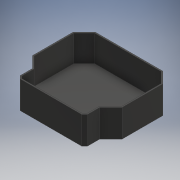
# Autodesk Inventor part: XT-SM-05
Saved by Autodesk Inventor 2017 (Build 210142000, 142)
## iProperties
Created: 2019-11-11
Part Number: XT-SM-05
Material: ABS Plastic
Document SubType Name: Modeling
Designer: Dell
Density: 1.06 g/cm^3
Appearance: Smooth - Black
Author: Dell
Autodesk Inventor part; units mm, degrees
ref_plane "YZ Plane" through (0, 0, 0) normal (1, 0, 0) x (0, 1, 0)
ref_plane "XZ Plane" through (0, 0, 0) normal (0, 1, 0) x (-1, 0, 0)
ref_plane "XY Plane" through (0, 0, 0) normal (0, 0, 1) x (1, 0, 0)
sketch "Sketch1" plane through (0, 0, 0) normal (0, 0, 1) x (1, 0, 0)
  line L0 (60.1273, -75.5) -> (55.1273, -80.5)
  line L1 (60.1273, -53.5) -> (60.1273, -75.5)
  line L2 (60.1273, -53.5) -> (80.1273, -33.5)
  line L3 (80.1273, 39) -> (80.1273, -33.5)
  line L4 (60.1273, 59) -> (80.1273, 39)
  line L5 (-60.1273, 59) -> (60.1273, 59)
  line L6 (-60.1273, 59) -> (-80.1273, 39)
  line L7 (-80.1273, 39) -> (-80.1273, -33.5)
  line L8 (-80.1273, -33.5) -> (-60.1273, -53.5)
  line L9 (-60.1273, -75.5) -> (-60.1273, -53.5)
  line L10 (-55.1273, -80.5) -> (-60.1273, -75.5)
  line L11 (55.1273, -80.5) -> (-55.1273, -80.5)
  point P0 (0, 0)
  point P1 (0, 0)
  point P2 (0, 59)
  dimension "d0" = 120.2547
  dimension "d1" = 72.5
  dimension "d2" = 22
  dimension "d3" = 110.2547
  dimension "d4" = 22
  dimension "d5" = 72.5
  dimension "d6" = 160.2547
  dimension "d7" = 139.5
  dimension "d8" = 27
  dimension "d9" = 27
  dimension "d10" = 20
  dimension "d11" = 20
  dimension "d12" = 20
  dimension "d14" = 20
  dimension "d15" = 20
  dimension "d16" = 5
  dimension "d17" = 20
  dimension "d18" = 59
  dimension "d19" = 80.1273
  constraints: 24 end point, 3 vertical, 1 coincident, 1 midpoint, 1 vertical alignment
  measures "d0" distance of L5.start L5.end
  measures "d1" distance of L4.end L2.end
  measures "d2" distance of L1.start L1.end
  measures "d3" distance of L11.start L10.start
  measures "d4" distance of L9.start L8.end
  measures "d5" distance of L7.start L8.start
  measures "d6" distance from line of L3 L7.start
  measures "d7" distance between parallel lines of L11 L5
  measures "d8" distance from line of L11 L8.end
  measures "d9" distance from line of L1.start L11
  measures "d10" distance from line of L7.start L5
  measures "d11" distance from line of L4.end L5
  measures "d12" horizontal distance of L8.start L8.end
  measures "d14" horizontal distance of L2.end L1.start
  measures "d15" horizontal distance of L2.end L1.start
  measures "d16" horizontal distance of L10.start L9.start
  measures "d17" horizontal distance of L5.start L7.start
  measures "d18" distance from line of L5 point (0, 0)
  measures "d19" distance from line of L7 point (0, 0)
extrude "Extrusion1" add sketch "Sketch1" along normal blind 2
sketch "Sketch2" plane through (0, 0, 2) normal (0, 0, 1) x (1, 0, 0)
  line L0 (-80.1273, 39) -> (-80.1273, -33.5) projected
  line L1 (-80.1273, -33.5) -> (-60.1273, -53.5) projected
  line L2 (-60.1273, -53.5) -> (-60.1273, -75.5) projected
  line L3 (-60.1273, -75.5) -> (-55.1273, -80.5) projected
  line L4 (-55.1273, -80.5) -> (55.1273, -80.5) projected
  line L5 (55.1273, -80.5) -> (60.1273, -75.5) projected
  line L6 (60.1273, -75.5) -> (60.1273, -53.5) projected
  line L7 (60.1273, -53.5) -> (80.1273, -33.5) projected
  line L8 (80.1273, -33.5) -> (80.1273, 39) projected
  line L9 (80.1273, 39) -> (60.1273, 59) projected
  line L10 (60.1273, 59) -> (-60.1273, 59) projected
  line L11 (-60.1273, 59) -> (-80.1273, 39) projected
  line L12 (-59.2575, 56.9) -> (59.2575, 56.9)
  line L13 (59.2575, 56.9) -> (78.0273, 38.1302)
  line L14 (78.0273, 38.1302) -> (78.0273, -32.6302)
  line L15 (78.0273, -32.6302) -> (58.0273, -52.6302)
  line L16 (58.0273, -52.6302) -> (58.0273, -74.6302)
  line L17 (58.0273, -74.6302) -> (54.2575, -78.4)
  line L18 (54.2575, -78.4) -> (-54.2575, -78.4)
  line L19 (-54.2575, -78.4) -> (-58.0273, -74.6302)
  line L20 (-58.0273, -74.6302) -> (-58.0273, -52.6302)
  line L21 (-58.0273, -52.6302) -> (-78.0273, -32.6302)
  line L22 (-78.0273, -32.6302) -> (-78.0273, 38.1302)
  line L23 (-78.0273, 38.1302) -> (-59.2575, 56.9)
  point P0 (0, 0)
  dimension "d22" = 2.1
  constraints: 24 end point, 11 other
  measures "d22" distance between parallel lines of L10 L12
extrude "Extrusion2" add sketch "Sketch2" along normal blind 47
body "Solid1"
